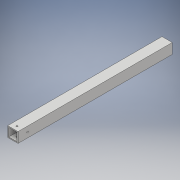
# Autodesk Inventor part: profile_alu
Saved by Autodesk Inventor 2017 (Build 210142000, 142)
## iProperties
Created: 2017-04-14
Part Number: profile_alu
Material: Generic
Document SubType Name: Modeling
Designer: franc
Density: 1 g/cm^3
Appearance: Default
Author: franc
Autodesk Inventor part; units mm, degrees
ref_plane "YZ Plane" through (0, 0, 0) normal (1, 0, 0) x (0, 1, 0)
ref_plane "XZ Plane" through (0, 0, 0) normal (0, 1, 0) x (-1, 0, 0)
ref_plane "XY Plane" through (0, 0, 0) normal (0, 0, 1) x (1, 0, 0)
sketch "Sketch1" plane through (0, 0, 0) normal (0, 1, 0) x (-1, 0, 0)
  line L0 (7.3913, 8.6413) -> (-12.6087, 8.6413)
  line L1 (-12.6087, 8.6413) -> (-12.6087, -11.3587)
  line L2 (-12.6087, -11.3587) -> (7.3913, -11.3587)
  line L3 (7.3913, -11.3587) -> (7.3913, 8.6413)
  line L4 (5.3913, 6.6413) -> (-10.6087, 6.6413)
  line L5 (-10.6087, 6.6413) -> (-10.6087, -9.3587)
  line L6 (-10.6087, -9.3587) -> (5.3913, -9.3587)
  line L7 (5.3913, -9.3587) -> (5.3913, 6.6413)
  point P0 (0, 0)
  dimension "d0" = 20
  dimension "d1" = 20
  dimension "d2" = 2
  dimension "d3" = 2
  dimension "d4" = 2
  dimension "d5" = 2
  constraints: 16 end point, 4 parallel, 2 horizontal, 2 perpendicular
  measures "d0" distance of L2.end L0.start
  measures "d1" distance of L0.start L0.end
  measures "d2" distance between parallel lines of L0 L4
  measures "d3" distance between parallel lines of L2 L6
  measures "d4" distance between parallel lines of L1 L5
  measures "d5" distance between parallel lines of L3 L7
extrude "Extrusion1" add sketch "Sketch1" along normal blind 300
sketch "Sketch2" plane through (-7.3913, 0, 8.6413) normal (0, 0, 1) x (1, 0, 0)
  circle A0 centre (10, 8) radius 1.5
  line L0 (0, 0) -> (0, 300) projected
  line L1 (0, 0) -> (20, 0) projected
  point P0 (7.3913, 0)
  dimension "d8" = 3
  dimension "d9" = 10
  dimension "d10" = 8
  constraints: 1 centre point
  measures "d8" diameter of A0
  measures "d9" distance from line of L0 A0.centre
  measures "d10" distance from line of L1 A0.centre
hole "Hole1" at (2.6087, 8, 8.6413) direction (0, 0, -1) diameter 3 end through all
sketch "Sketch3" plane through (-7.3913, 0, -11.3587) normal (-1, 0, 0) x (0, 0, 1)
  circle A0 centre (10, 18.5) radius 1.5
  line L0 (0, 0) -> (20, 0) projected
  line L1 (0, 0) -> (0, 300) projected
  point P0 (11.3587, 0)
  dimension "d18" = 18.5
  dimension "d19" = 10
  dimension "d20" = 3
  constraints: 1 centre point
  measures "d18" distance from line of L0 A0.centre
  measures "d19" distance from line of L1 A0.centre
  measures "d20" diameter of A0
hole "Hole2" at (-7.3913, 18.5, -1.3587) direction (1, 0, 0) diameter 3 end through all
body "Solid1"
